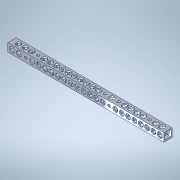
# Autodesk Inventor part: ロボット回転9x9_3
Saved by Autodesk Inventor 2020.3 (Build 243373000, 373)
## iProperties
Created: 2020-07-05
Part Number: ロボット回転9x9_3
Material: アルミニウム 6061
Document SubType Name: Modeling
Designer: totot
Density: 2.7 g/cm^3
Appearance: アルミニウム - フラット
Mass: 16.4941 g
Surface Area: 104.826 cm^2
Volume: 6.10894 cm^3
Author: totot
Autodesk Inventor part; units mm, degrees
ref_plane "YZ Plane" through (0, 0, 0) normal (1, 0, 0) x (0, 1, 0)
ref_plane "XZ Plane" through (0, 0, 0) normal (0, 1, 0) x (-1, 0, 0)
ref_plane "XY Plane" through (0, 0, 0) normal (0, 0, 1) x (1, 0, 0)
sketch "スケッチ1" plane through (0, 0, 0) normal (1, 0, 0) x (0, 1, 0)
  line L0 (0, 0) -> (9, 0)
  line L1 (9, 0) -> (9, 9)
  line L2 (9, 9) -> (0, 9)
  line L3 (0, 9) -> (0, 0)
  line L4 (1.2, 7.8) -> (7.8, 7.8)
  line L5 (7.8, 7.8) -> (7.8, 1.2)
  line L6 (7.8, 1.2) -> (1.2, 1.2)
  line L7 (1.2, 1.2) -> (1.2, 7.8)
  dimension "d0" = 9
  dimension "d1" = 9
  dimension "d2" = 6.6
  dimension "d3" = 6.6
  dimension "d4" = 1.2
  dimension "d5" = 1.2
  constraints: 16 end point, 4 parallel, 2 horizontal, 2 perpendicular
  measures "d0" distance of L2.end L1.end
  measures "d1" distance of L1.end L0.end
  measures "d2" distance of L5.end L6.end
  measures "d3" distance of L6.end L4.start
  measures "d4" distance between parallel lines of L0 L6
  measures "d5" distance between parallel lines of L7 L3
extrude "押し出し1" add sketch "スケッチ1" along normal blind 99.5097
sketch "スケッチ2" plane through (0, 0, 9) normal (0, 0, 1) x (1, 0, 0)
  line L0 (0, 9) -> (0, 0) projected
  line L1 (0, 9) -> (99.5097, 9) projected
  line L2 (99.5097, 9) -> (99.5097, 0) projected
  point P0 (4.5, 4.5)
  point P1 (95.0097, 4.5)
  dimension "d8" = 4.5
  dimension "d9" = 4.5
  dimension "d10" = 4.5
  dimension "d11" = 4.5
  measures "d8" distance from line of point (4.5, 4.5) L0
  measures "d9" distance from line of point (4.5, 4.5) L1
  measures "d10" distance from line of L2 point (95.01, 4.5)
  measures "d11" distance from line of L1 point (95.01, 4.5)
hole "穴1" at (4.5, 4.5, 9) at (95.0097, 4.5, 9) direction (0, 0, -1) diameter 3 end through all
sketch "スケッチ3" plane through (0, 9, 9) normal (0, 1, 0) x (1, 0, 0)
  line L0 (0, 0) -> (99.5097, 0) projected
  line L1 (0, 9) -> (0, 0) projected
  line L2 (99.5097, 9) -> (99.5097, 0) projected
  point P0 (13.5, 4.5)
  point P1 (86.0097, 4.5)
  dimension "d19" = 4.5
  dimension "d20" = 13.5
  dimension "d21" = 13.5
  dimension "d22" = 4.5
  measures "d19" distance from line of point (13.5, 4.5) L0
  measures "d20" distance from line of point (13.5, 4.5) L1
  measures "d21" distance from line of L2 point (86.01, 4.5)
  measures "d22" distance from line of L0 point (86.01, 4.5)
hole "穴2" at (13.5, 9, 4.5) at (86.0097, 9, 4.5) direction (0, -1, 0) diameter 3 end through all
sketch "スケッチ4" plane through (99.5097, 0, 0) normal (1, 0, 0) x (0, 0, -1)
  line L0 (0, 9) -> (-9, 9) projected
  line L1 (0, 0) -> (-9, 0)
  line L2 (-9, 0) -> (-9, 9)
  line L3 (-9, 9) -> (0, 9)
  line L4 (0, 9) -> (0, 0)
  line L5 (-1.2, 1.2) -> (-7.8, 1.2) projected
  line L6 (-7.8, 1.2) -> (-7.8, 7.8) projected
  line L7 (-1.2, 1.2) -> (-7.8, 1.2)
  line L8 (-7.8, 1.2) -> (-7.8, 7.8)
  line L9 (-7.8, 7.8) -> (-1.2, 7.8)
  line L10 (-1.2, 7.8) -> (-1.2, 1.2)
  dimension "d30" = 6.6
  dimension "d31" = 6.6
  constraints: 16 end point, 4 parallel, 2 horizontal, 2 perpendicular
  measures "d30" distance of L6.end L9.end
  measures "d31" distance of L7.end L6.end
extrude "押し出し2" add sketch "スケッチ4" along normal blind 55
sketch "スケッチ5" plane through (0, 0, 0) normal (-1, 0, 0) x (0, 0, 1)
  line L0 (0, 9) -> (9, 9) projected
  line L1 (0, 0) -> (9, 0)
  line L2 (9, 0) -> (9, 9)
  line L3 (9, 9) -> (0, 9)
  line L4 (0, 9) -> (0, 0)
  line L5 (1.2, 1.2) -> (7.8, 1.2) projected
  line L6 (7.8, 1.2) -> (7.8, 7.8) projected
  line L7 (1.2, 1.2) -> (7.8, 1.2)
  line L8 (7.8, 1.2) -> (7.8, 7.8)
  line L9 (7.8, 7.8) -> (1.2, 7.8)
  line L10 (1.2, 7.8) -> (1.2, 1.2)
  constraints: 16 end point, 4 parallel, 2 horizontal, 2 perpendicular
extrude "押し出し3" add sketch "スケッチ5" along normal blind 15
sketch "スケッチ6" plane through (154.5097, 0, 0) normal (0, 0, -1) x (-1, 0, 0)
  line L0 (169.5097, 9) -> (169.5097, 0) projected
  line L1 (0, 9) -> (169.5097, 9) projected
  line L2 (0, 0) -> (0, 9) projected
  point P0 (154.5097, 0)
  point P1 (165.0097, 4.5)
  point P2 (4.5, 4.5)
  dimension "d36" = 4.5
  dimension "d37" = 4.5
  dimension "d38" = 4.5
  dimension "d39" = 4.5
  measures "d36" distance from line of point (165.01, 4.5) L0
  measures "d37" distance from line of point (165.01, 4.5) L1
  measures "d38" distance from line of L1 point (4.5, 4.5)
  measures "d39" distance from line of point (4.5, 4.5) L2
hole "穴3" at (-10.5, 4.5, 0) at (150.0097, 4.5, 0) direction (0, 0, 1) diameter 6 end through all
sketch "スケッチ7" plane through (154.5097, 9, 9) normal (0, 1, 0) x (1, 0, 0)
  line L0 (0, 9) -> (0, 0) projected
  circle A0 centre (-68.5, 4.5) radius 1.5 projected
  line L1 (0, 9) -> (-169.5097, 9) projected
  point P0 (-154.5097, 9)
  point P1 (-53.5, 4.5)
  point P2 (-20, 4.5)
  dimension "d47" = 20
  dimension "d48" = 15
  dimension "d49" = 4.5
  dimension "d50" = 4.5
  measures "d47" distance from line of point (-20, 4.5) L0
  measures "d48" distance of point (-53.5, 4.5) A0.centre
  measures "d49" distance from line of point (-53.5, 4.5) L1
  measures "d50" distance from line of point (-20, 4.5) L1
hole "穴4" at (101.0097, 9, 4.5) at (134.5097, 9, 4.5) direction (0, -1, 0) diameter 3 end through all
sketch "スケッチ8" plane through (154.5097, 9, 9) normal (0, 1, 0) x (1, 0, 0)
  line L0 (-169.5097, 0) -> (-169.5097, 9) projected
  circle A0 centre (-141.0097, 4.5) radius 1.5 projected
  line L1 (0, 9) -> (-169.5097, 9) projected
  circle A1 centre (-68.5, 4.5) radius 1.5 projected
  circle A2 centre (-68.5, 4.5) radius 1.5 projected
  line L2 (-141.0097, 4.5) -> (-68.5, 4.5)
  circle A3 centre (-53.5, 4.5) radius 1.5 projected
  circle A4 centre (-20, 4.5) radius 1.5 projected
  line L3 (0, 9) -> (0, 0) projected
  point P0 (-154.5097, 9)
  point P1 (-162.3847, 4.5)
  point P2 (-155.2597, 4.5)
  point P3 (-148.1347, 4.5)
  point P4 (-134.4179, 4.5)
  point P5 (-127.8261, 4.5)
  point P6 (-121.2343, 4.5)
  point P7 (-114.6425, 4.5)
  point P8 (-108.0507, 4.5)
  point P9 (-101.4589, 4.5)
  point P10 (-94.8672, 4.5)
  point P11 (-88.2754, 4.5)
  point P12 (-81.6836, 4.5)
  point P13 (-75.0918, 4.5)
  point P14 (-61, 4.5)
  point P15 (-46.8, 4.5)
  point P16 (-40.1, 4.5)
  point P17 (-33.4, 4.5)
  point P18 (-26.7, 4.5)
  point P19 (-13.3333, 4.5)
  point P20 (-6.6667, 4.5)
  dimension "d58" = 28.5
  dimension "d59" = 7.125
  dimension "d60" = 4.5
  dimension "d63" = 7.125
  dimension "d68" = 72.5097
  dimension "d69" = 6.5918
  dimension "d72" = 6.5918
  dimension "d77" = 15
  dimension "d78" = 7.5
  dimension "d79" = 4.5
  dimension "d80" = 33.5
  dimension "d81" = 4.5
  dimension "d82" = 6.7
  dimension "d85" = 6.7
  dimension "d90" = 20
  dimension "d91" = 4.5
  dimension "d92" = 6.6667
  dimension "d95" = 6.6667
  constraints: 5 horizontal, 2 end point, 1 point on line, 15 other
  measures "d58" distance from line of L0 L2.start
  measures "d59" distance from line of point (-162.385, 4.5) L0
  measures "d60" distance from line of point (-162.385, 4.5) L1
  measures "d63" distance of point (-162.385, 4.5) point (-155.26, 4.5)
  measures "d68" distance of L2.start A1.centre
  measures "d69" distance of L2.start point (-134.418, 4.5)
  measures "d72" distance of point (-134.418, 4.5) point (-127.826, 4.5)
  measures "d77" distance of A1.centre A3.centre
  measures "d78" distance of A1.centre point (-61, 4.5)
  measures "d79" distance from line of point (-61, 4.5) L1
  measures "d80" distance of A3.centre A4.centre
  measures "d81" distance from line of point (-46.8, 4.5) L1
  measures "d82" distance of point (-46.8, 4.5) A3.centre
  measures "d85" distance of point (-46.8, 4.5) point (-40.1, 4.5)
  measures "d90" distance from line of A4.centre L3
  measures "d91" distance from line of point (-13.333, 4.5) L1
  measures "d92" distance of point (-13.333, 4.5) A4.centre
  measures "d95" distance of point (-13.333, 4.5) point (-6.667, 4.5)
hole "穴5" at (-7.875, 9, 4.5) at (-0.75, 9, 4.5) at (6.375, 9, 4.5) at (20.0918, 9, 4.5) at (26.6836, 9, 4.5) at (33.2754, 9, 4.5) at (39.8672, 9, 4.5) at (46.4589, 9, 4.5) at (53.0507, 9, 4.5) at (59.6425, 9, 4.5) at (66.2343, 9, 4.5) at (72.8261, 9, 4.5) at (79.4179, 9, 4.5) at (93.5097, 9, 4.5) at (107.7097, 9, 4.5) at (114.4097, 9, 4.5) at (121.1097, 9, 4.5) at (127.8097, 9, 4.5) at (141.1763, 9, 4.5) at (147.843, 9, 4.5) direction (0, -1, 0) diameter 5.5 end through all
sketch "スケッチ9" plane through (154.5097, 0, 0) normal (0, 0, -1) x (-1, 0, 0)
  circle A0 centre (59.5, 4.5) radius 1.5 projected
  circle A1 centre (150.0097, 4.5) radius 1.5 projected
  line L0 (0, 9) -> (169.5097, 9) projected
  circle A2 centre (4.5, 4.5) radius 3 projected
  point P0 (154.5097, 0)
  point P1 (66.4623, 4.5)
  point P2 (73.4246, 4.5)
  point P3 (80.3868, 4.5)
  point P4 (87.3491, 4.5)
  point P5 (94.3114, 4.5)
  point P6 (101.2737, 4.5)
  point P7 (108.236, 4.5)
  point P8 (115.1983, 4.5)
  point P9 (122.1605, 4.5)
  point P10 (129.1228, 4.5)
  point P11 (136.0851, 4.5)
  point P12 (143.0474, 4.5)
  point P13 (11.375, 4.5)
  point P14 (18.25, 4.5)
  point P15 (25.125, 4.5)
  point P16 (32, 4.5)
  point P17 (38.875, 4.5)
  point P18 (45.75, 4.5)
  point P19 (52.625, 4.5)
  dimension "d107" = 87.5097
  dimension "d108" = 90.5097
  dimension "d109" = 4.5
  dimension "d110" = 6.9623
  dimension "d113" = 6.9623
  dimension "d118" = 55
  dimension "d119" = 4.5
  dimension "d120" = 6.875
  dimension "d123" = 6.875
  constraints: 2 horizontal, 17 other
  measures "d108" distance of A0.centre A1.centre
  measures "d109" distance from line of L0 point (66.462, 4.5)
  measures "d110" distance of point (66.462, 4.5) A0.centre
  measures "d113" distance of point (66.462, 4.5) point (73.425, 4.5)
  measures "d118" distance of A0.centre A2.centre
  measures "d119" distance from line of L0 point (11.375, 4.5)
  measures "d120" distance of point (11.375, 4.5) A2.centre
  measures "d123" distance of point (11.375, 4.5) point (18.25, 4.5)
hole "穴6" at (88.0474, 4.5, 0) at (81.0851, 4.5, 0) at (74.1228, 4.5, 0) at (67.1605, 4.5, 0) at (60.1983, 4.5, 0) at (53.236, 4.5, 0) at (46.2737, 4.5, 0) at (39.3114, 4.5, 0) at (32.3491, 4.5, 0) at (25.3868, 4.5, 0) at (18.4246, 4.5, 0) at (11.4623, 4.5, 0) at (143.1347, 4.5, 0) at (136.2597, 4.5, 0) at (129.3847, 4.5, 0) at (122.5097, 4.5, 0) at (115.6347, 4.5, 0) at (108.7597, 4.5, 0) at (101.8847, 4.5, 0) direction (0, 0, 1) diameter 5.5 end through all
sketch "スケッチ10" plane through (154.5097, 0, 0) normal (0, 0, -1) x (-1, 0, 0)
  line L0 (169.5097, 0) -> (0, 0) projected
  circle A0 centre (165.0097, 4.5) radius 3 projected
  circle A1 centre (150.0097, 4.5) radius 1.5 projected
  point P0 (154.5097, 0)
  point P1 (157.5097, 4.5)
  dimension "d135" = 4.5
  dimension "d136" = 15
  dimension "d137" = 7.5
  measures "d135" distance from line of L0 point (157.51, 4.5)
  measures "d136" distance of A0.centre A1.centre
  measures "d137" distance of point (157.51, 4.5) A1.centre
hole "穴7" at (-3, 4.5, 0) direction (0, 0, 1) diameter 5.5 end through all
equation "\"d3\" = d2"
equation "\"d5\" = d4"
equation "\"d9\" = d8"
equation "\"d37\" = d36"
equation "\"d38\" = d36"
equation "\"d39\" = d38"
equation "\"d50\" = d49"
equation "\"d59\" = 0.25 * d58"
equation "\"d63\" = d59"
equation "\"d69\" = 0.0909091 * d68"
equation "\"d72\" = d69"
equation "\"d78\" = 0.5 * d77"
equation "\"d81\" = d79"
equation "\"d82\" = 0.2 * d80"
equation "\"d85\" = d82"
equation "\"d92\" = 0.333333 * d90"
equation "\"d95\" = d92"
equation "\"d110\" = 0.0769231 * d108"
equation "\"d113\" = d110"
equation "\"d120\" = 0.125 * d118"
equation "\"d123\" = d120"
equation "\"d137\" = 0.5 * d136"
